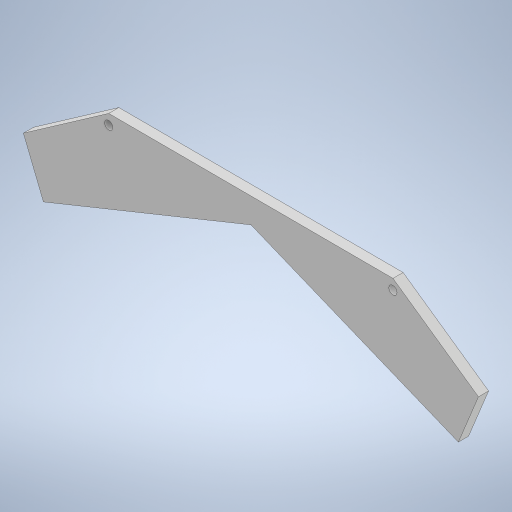
# Autodesk Inventor part: zaver
Saved by Autodesk Inventor 2024 (Build 280153000, 153)
## iProperties
Created: 2024-03-06
Part Number: zaver
Material: Všeobecné
Document SubType Name: Modeling
Designer: Game
Density: 1 g/cm^3
Appearance: Výchozí
Author: Game
Autodesk Inventor part; units mm, degrees
ref_plane "YZ Plane" through (0, 0, 0) normal (1, 0, 0) x (0, 1, 0)
ref_plane "XZ Plane" through (0, 0, 0) normal (0, 1, 0) x (-1, 0, 0)
ref_plane "XY Plane" through (0, 0, 0) normal (0, 0, 1) x (1, 0, 0)
sketch "Náčrt1" plane through (0, 0, 0) normal (0, 0, 1) x (1, 0, 0)
  line L0 (70.5158, 9.6388) -> (-69.4838, 10)
  line L1 (70.5158, 9.6388) -> (137.3455, -37.1558)
  line L2 (70.5158, 9.6388) -> (152.0998, 9.6388) construction
  line L3 (137.3455, -37.1558) -> (125.874, -53.5389)
  line L4 (-69.4838, 10) -> (-136.3135, -36.7947)
  line L5 (-69.4838, 10) -> (12.1002, 10) construction
  line L6 (-136.3135, -36.7947) -> (-124.8419, -53.1777)
  line L7 (0.6215, 10) -> (0.5893, -2.5)
  line L8 (-124.8419, -53.1777) -> (0.5893, -2.5)
  line L9 (125.874, -53.5389) -> (0.5893, -2.5)
  point P0 (0, 0)
  dimension "d2" = 140
  dimension "d3" = 81.584
  dimension "d4" = 35
  dimension "d5" = 20
  dimension "d6" = 81.584
  dimension "d7" = 145
  dimension "d8" = 20
  dimension "d9" = 12.5
  dimension "d22" = 135.282
  dimension "d23" = 135.282
  constraints: 20 end point, 3 perpendicular, 2 equal length, 2 horizontal, 1 point on line
  measures "d2" distance of L0.start L0.end
  measures "d3" distance of L0.start L1.end
  measures "d4" angle of L1 L2
  measures "d5" distance of L1.end L3.end
  measures "d6" distance of L0.end L4.end
  measures "d7" angle of L4 L5
  measures "d8" distance of L4.end L6.end
  measures "d9" distance of L7.start L7.end
  measures "d22" distance of L6.end L7.end
  measures "d23" distance of L3.end L7.end
extrude "Vysunutí1" add sketch "Náčrt1" along normal blind 5
sketch "Náčrt2" plane through (0, 0, 5) normal (0, 0, 1) x (1, 0, 0)
  line L0 (-136.3135, -36.7947) -> (-124.8419, -53.1777) projected
  line L1 (-124.8419, -53.1777) -> (-101.6623, -43.8125)
  line L2 (-124.8419, -53.1777) -> (0.5893, -2.5) projected
  line L3 (-101.6623, -43.8125) -> (-111.5137, -19.4297)
  line L4 (-69.4838, 10) -> (-136.3135, -36.7947) projected
  line L5 (-136.3135, -36.7947) -> (-124.8419, -53.1777)
  line L6 (0.5893, -2.5) -> (125.874, -53.5389) projected
  line L7 (125.874, -53.5389) -> (102.7215, -44.1069)
  line L8 (102.7215, -44.1069) -> (112.6093, -19.8353)
  line L9 (137.3455, -37.1558) -> (70.5158, 9.6388) projected
  line L10 (137.3455, -37.1558) -> (112.6093, -19.8353)
  line L11 (125.874, -53.5389) -> (137.3455, -37.1558) projected
  line L12 (125.874, -53.5389) -> (137.3455, -37.1558)
  point P0 (0, 0)
  dimension "d12" = 25
  dimension "d13" = 25
  constraints: 14 end point, 4 point on line, 3 perpendicular, 2 collinear
  measures "d12" distance of L0.end L1.end
  measures "d13" distance of L6.end L7.end
extrude "Vysunutí2" cut sketch "Náčrt2" against normal blind 5
sketch "Náčrt5" plane through (0, 0, 5) normal (0, 0, 1) x (1, 0, 0)
  line L0 (70.5158, 9.6388) -> (-69.4838, 10) projected
  line L1 (-69.4838, 10) -> (-69.4838, 5)
  line L2 (-69.4838, 10) -> (-64.4838, 10) construction
  line L3 (112.6093, -19.8353) -> (70.5158, 9.6388) projected
  line L4 (70.5158, 9.6388) -> (70.5158, 4.6388)
  line L5 (70.5158, 9.6388) -> (75.5158, 9.6388) construction
  circle A0 centre (-69.4838, 5) radius 2
  circle A1 centre (70.5158, 4.6388) radius 2
  point P0 (0, 0)
  dimension "d24" = 5
  dimension "d25" = 90
  dimension "d26" = 5
  dimension "d27" = 90
  dimension "d28" = 4
  dimension "d29" = 4
  constraints: 8 end point, 2 centre point, 2 coincident, 2 horizontal, 2 perpendicular, 2 vertical
  measures "d24" distance of L0.end L1.end
  measures "d25" angle of L1 L2
  measures "d26" distance of L0.start L4.end
  measures "d27" angle of L4 L5
  measures "d28" diameter of A0
  measures "d29" diameter of A1
extrude "Vysunutí4" cut sketch "Náčrt5" against normal blind 10
